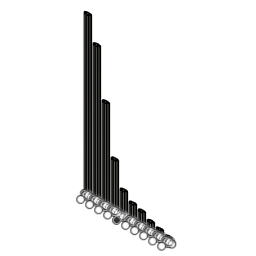
TT Clips 2020 v5 (Autodesk Fusion 360 design; units mm, degrees)
Autodesk Fusion 360 part; units mm, degrees
other "Mesh1"
sketch "Sketch1" plane through (0, 0, 0) normal (0, 0, 1) x (1, 0, 0)
  line L0 (-7.5, -1.2) -> (-7.5, 0)
  arc A0 (3.2, 0) -> (2, -1.2) centre (3.2, -1.2) ccw
  line L1 (3.2, -1.2) -> (7.5, -1.2)
  arc A1 (-6.7104, 1.1276) -> (-7.5, 0) centre (-6.3, 0) ccw
  line L2 (-2, -1.2) -> (-2, -4.3798)
  line L3 (2, -1.2) -> (2, -4.3798)
  arc A2 (-3.2, -3.4) -> (-2, -4.3798) centre (-3, -4.3798) ccw
  line L4 (-3.2, -3.4) -> (-3.2, -1.2)
  arc A3 (7.5, 0) -> (6.7104, 1.1276) centre (6.3, 0) ccw
  arc A4 (2, -4.3798) -> (3.2, -3.4) centre (3, -4.3798) ccw
  line L5 (7.5, -1.2) -> (7.5, 0)
  line L6 (6.3, 0) -> (3.2, 0)
  arc A5 (-2, -1.2) -> (-3.2, 0) centre (-3.2, -1.2) ccw
  line L7 (0, -6.5) -> (0, 3.9) construction
  line L8 (-3.2, -1.2) -> (-7.5, -1.2)
  line L9 (3.2, -3.4) -> (3.2, -1.2)
  line L10 (-6.3, 0) -> (-3.2, 0)
  arc A6 (6.7104, 1.1276) -> (-6.7104, 1.1276) centre (0, -17.3091) ccw
  arc A7 (6.3, 0) -> (-6.3, 0) centre (0, -16.1091) ccw
  line L11 (-80, -6.5) -> (-80, 3.9) construction
  arc A8 (-76.8, 0) -> (-78, -1.2) centre (-76.8, -1.2) ccw
  line L12 (-83.2, -3.4) -> (-83.2, -1.2)
  line L13 (-72.5, -1.2) -> (-72.5, 0)
  line L14 (-76.8, -3.4) -> (-76.8, -1.2)
  line L15 (-87.5, -1.2) -> (-87.5, 0)
  arc A9 (-78, -4.3798) -> (-76.8, -3.4) centre (-77, -4.3798) ccw
  line L16 (-82, -1.2) -> (-82, -4.3798)
  arc A10 (-86.7104, 1.1276) -> (-87.5, 0) centre (-86.3, 0) ccw
  line L17 (-86.3, 0) -> (-83.2, 0)
  line L18 (-78, -1.2) -> (-78, -4.3798)
  arc A11 (-82, -1.2) -> (-83.2, 0) centre (-83.2, -1.2) ccw
  arc A12 (-83.2, -3.4) -> (-82, -4.3798) centre (-83, -4.3798) ccw
  line L19 (-83.2, -1.2) -> (-87.5, -1.2)
  line L20 (-73.7, 0) -> (-76.8, 0)
  arc A13 (-73.2896, 1.1276) -> (-86.7104, 1.1276) centre (-80, -17.3091) ccw
  arc A14 (-73.7, 0) -> (-86.3, 0) centre (-80, -16.1091) ccw
  line L21 (-76.8, -1.2) -> (-72.5, -1.2)
  arc A15 (-72.5, 0) -> (-73.2896, 1.1276) centre (-73.7, 0) ccw
  line L22 (-60, -6.5) -> (-60, 3.9) construction
  arc A16 (-56.8, 0) -> (-58, -1.2) centre (-56.8, -1.2) ccw
  line L23 (-63.2, -3.4) -> (-63.2, -1.2)
  line L24 (-52.5, -1.2) -> (-52.5, 0)
  line L25 (-56.8, -3.4) -> (-56.8, -1.2)
  line L26 (-67.5, -1.2) -> (-67.5, 0)
  arc A17 (-58, -4.3798) -> (-56.8, -3.4) centre (-57, -4.3798) ccw
  line L27 (-62, -1.2) -> (-62, -4.3798)
  arc A18 (-66.7104, 1.1276) -> (-67.5, 0) centre (-66.3, 0) ccw
  line L28 (-66.3, 0) -> (-63.2, 0)
  line L29 (-58, -1.2) -> (-58, -4.3798)
  arc A19 (-62, -1.2) -> (-63.2, 0) centre (-63.2, -1.2) ccw
  arc A20 (-63.2, -3.4) -> (-62, -4.3798) centre (-63, -4.3798) ccw
  line L30 (-63.2, -1.2) -> (-67.5, -1.2)
  line L31 (-53.7, 0) -> (-56.8, 0)
  arc A21 (-53.2896, 1.1276) -> (-66.7104, 1.1276) centre (-60, -17.3091) ccw
  arc A22 (-53.7, 0) -> (-66.3, 0) centre (-60, -16.1091) ccw
  line L32 (-56.8, -1.2) -> (-52.5, -1.2)
  arc A23 (-52.5, 0) -> (-53.2896, 1.1276) centre (-53.7, 0) ccw
  line L33 (-40, -6.5) -> (-40, 3.9) construction
  arc A24 (-36.8, 0) -> (-38, -1.2) centre (-36.8, -1.2) ccw
  line L34 (-43.2, -3.4) -> (-43.2, -1.2)
  line L35 (-32.5, -1.2) -> (-32.5, 0)
  line L36 (-36.8, -3.4) -> (-36.8, -1.2)
  line L37 (-47.5, -1.2) -> (-47.5, 0)
  arc A25 (-38, -4.3798) -> (-36.8, -3.4) centre (-37, -4.3798) ccw
  line L38 (-42, -1.2) -> (-42, -4.3798)
  arc A26 (-46.7104, 1.1276) -> (-47.5, 0) centre (-46.3, 0) ccw
  line L39 (-46.3, 0) -> (-43.2, 0)
  line L40 (-38, -1.2) -> (-38, -4.3798)
  arc A27 (-42, -1.2) -> (-43.2, 0) centre (-43.2, -1.2) ccw
  arc A28 (-43.2, -3.4) -> (-42, -4.3798) centre (-43, -4.3798) ccw
  line L41 (-43.2, -1.2) -> (-47.5, -1.2)
  line L42 (-33.7, 0) -> (-36.8, 0)
  arc A29 (-33.2896, 1.1276) -> (-46.7104, 1.1276) centre (-40, -17.3091) ccw
  arc A30 (-33.7, 0) -> (-46.3, 0) centre (-40, -16.1091) ccw
  line L43 (-36.8, -1.2) -> (-32.5, -1.2)
  arc A31 (-32.5, 0) -> (-33.2896, 1.1276) centre (-33.7, 0) ccw
  line L44 (-20, -6.5) -> (-20, 3.9) construction
  arc A32 (-16.8, 0) -> (-18, -1.2) centre (-16.8, -1.2) ccw
  line L45 (-23.2, -3.4) -> (-23.2, -1.2)
  line L46 (-12.5, -1.2) -> (-12.5, 0)
  line L47 (-16.8, -3.4) -> (-16.8, -1.2)
  line L48 (-27.5, -1.2) -> (-27.5, 0)
  arc A33 (-18, -4.3798) -> (-16.8, -3.4) centre (-17, -4.3798) ccw
  line L49 (-22, -1.2) -> (-22, -4.3798)
  arc A34 (-26.7104, 1.1276) -> (-27.5, 0) centre (-26.3, 0) ccw
  line L50 (-26.3, 0) -> (-23.2, 0)
  line L51 (-18, -1.2) -> (-18, -4.3798)
  arc A35 (-22, -1.2) -> (-23.2, 0) centre (-23.2, -1.2) ccw
  arc A36 (-23.2, -3.4) -> (-22, -4.3798) centre (-23, -4.3798) ccw
  line L52 (-23.2, -1.2) -> (-27.5, -1.2)
  line L53 (-13.7, 0) -> (-16.8, 0)
  arc A37 (-13.2896, 1.1276) -> (-26.7104, 1.1276) centre (-20, -17.3091) ccw
  arc A38 (-13.7, 0) -> (-26.3, 0) centre (-20, -16.1091) ccw
  line L54 (-16.8, -1.2) -> (-12.5, -1.2)
  arc A39 (-12.5, 0) -> (-13.2896, 1.1276) centre (-13.7, 0) ccw
  line L55 (20, -6.5) -> (20, 3.9) construction
  arc A40 (23.2, 0) -> (22, -1.2) centre (23.2, -1.2) ccw
  line L56 (16.8, -3.4) -> (16.8, -1.2)
  line L57 (27.5, -1.2) -> (27.5, 0)
  line L58 (23.2, -3.4) -> (23.2, -1.2)
  line L59 (12.5, -1.2) -> (12.5, 0)
  arc A41 (22, -4.3798) -> (23.2, -3.4) centre (23, -4.3798) ccw
  line L60 (18, -1.2) -> (18, -4.3798)
  arc A42 (13.2896, 1.1276) -> (12.5, 0) centre (13.7, 0) ccw
  line L61 (13.7, 0) -> (16.8, 0)
  line L62 (22, -1.2) -> (22, -4.3798)
  arc A43 (18, -1.2) -> (16.8, 0) centre (16.8, -1.2) ccw
  arc A44 (16.8, -3.4) -> (18, -4.3798) centre (17, -4.3798) ccw
  line L63 (16.8, -1.2) -> (12.5, -1.2)
  line L64 (26.3, 0) -> (23.2, 0)
  arc A45 (26.7104, 1.1276) -> (13.2896, 1.1276) centre (20, -17.3091) ccw
  arc A46 (26.3, 0) -> (13.7, 0) centre (20, -16.1091) ccw
  line L65 (23.2, -1.2) -> (27.5, -1.2)
  arc A47 (27.5, 0) -> (26.7104, 1.1276) centre (26.3, 0) ccw
  line L66 (40, -6.5) -> (40, 3.9) construction
  arc A48 (43.2, 0) -> (42, -1.2) centre (43.2, -1.2) ccw
  line L67 (36.8, -3.4) -> (36.8, -1.2)
  line L68 (47.5, -1.2) -> (47.5, 0)
  line L69 (43.2, -3.4) -> (43.2, -1.2)
  line L70 (32.5, -1.2) -> (32.5, 0)
  arc A49 (42, -4.3798) -> (43.2, -3.4) centre (43, -4.3798) ccw
  line L71 (38, -1.2) -> (38, -4.3798)
  arc A50 (33.2896, 1.1276) -> (32.5, 0) centre (33.7, 0) ccw
  line L72 (33.7, 0) -> (36.8, 0)
  line L73 (42, -1.2) -> (42, -4.3798)
  arc A51 (38, -1.2) -> (36.8, 0) centre (36.8, -1.2) ccw
  arc A52 (36.8, -3.4) -> (38, -4.3798) centre (37, -4.3798) ccw
  line L74 (36.8, -1.2) -> (32.5, -1.2)
  line L75 (46.3, 0) -> (43.2, 0)
  arc A53 (46.7104, 1.1276) -> (33.2896, 1.1276) centre (40, -17.3091) ccw
  arc A54 (46.3, 0) -> (33.7, 0) centre (40, -16.1091) ccw
  line L76 (43.2, -1.2) -> (47.5, -1.2)
  arc A55 (47.5, 0) -> (46.7104, 1.1276) centre (46.3, 0) ccw
  line L77 (60, -6.5) -> (60, 3.9) construction
  arc A56 (63.2, 0) -> (62, -1.2) centre (63.2, -1.2) ccw
  line L78 (56.8, -3.4) -> (56.8, -1.2)
  line L79 (67.5, -1.2) -> (67.5, 0)
  line L80 (63.2, -3.4) -> (63.2, -1.2)
  line L81 (52.5, -1.2) -> (52.5, 0)
  arc A57 (62, -4.3798) -> (63.2, -3.4) centre (63, -4.3798) ccw
  line L82 (58, -1.2) -> (58, -4.3798)
  arc A58 (53.2896, 1.1276) -> (52.5, 0) centre (53.7, 0) ccw
  line L83 (53.7, 0) -> (56.8, 0)
  line L84 (62, -1.2) -> (62, -4.3798)
  arc A59 (58, -1.2) -> (56.8, 0) centre (56.8, -1.2) ccw
  arc A60 (56.8, -3.4) -> (58, -4.3798) centre (57, -4.3798) ccw
  line L85 (56.8, -1.2) -> (52.5, -1.2)
  line L86 (66.3, 0) -> (63.2, 0)
  arc A61 (66.7104, 1.1276) -> (53.2896, 1.1276) centre (60, -17.3091) ccw
  arc A62 (66.3, 0) -> (53.7, 0) centre (60, -16.1091) ccw
  line L87 (63.2, -1.2) -> (67.5, -1.2)
  arc A63 (67.5, 0) -> (66.7104, 1.1276) centre (66.3, 0) ccw
  line L88 (80, -6.5) -> (80, 3.9) construction
  arc A64 (83.2, 0) -> (82, -1.2) centre (83.2, -1.2) ccw
  line L89 (76.8, -3.4) -> (76.8, -1.2)
  line L90 (87.5, -1.2) -> (87.5, 0)
  line L91 (83.2, -3.4) -> (83.2, -1.2)
  line L92 (72.5, -1.2) -> (72.5, 0)
  arc A65 (82, -4.3798) -> (83.2, -3.4) centre (83, -4.3798) ccw
  line L93 (78, -1.2) -> (78, -4.3798)
  arc A66 (73.2896, 1.1276) -> (72.5, 0) centre (73.7, 0) ccw
  line L94 (73.7, 0) -> (76.8, 0)
  line L95 (82, -1.2) -> (82, -4.3798)
  arc A67 (78, -1.2) -> (76.8, 0) centre (76.8, -1.2) ccw
  arc A68 (76.8, -3.4) -> (78, -4.3798) centre (77, -4.3798) ccw
  line L96 (76.8, -1.2) -> (72.5, -1.2)
  line L97 (86.3, 0) -> (83.2, 0)
  arc A69 (86.7104, 1.1276) -> (73.2896, 1.1276) centre (80, -17.3091) ccw
  arc A70 (86.3, 0) -> (73.7, 0) centre (80, -16.1091) ccw
  line L98 (83.2, -1.2) -> (87.5, -1.2)
  arc A71 (87.5, 0) -> (86.7104, 1.1276) centre (86.3, 0) ccw
  line L99 (100, -6.5) -> (100, 3.9) construction
  arc A72 (103.2, 0) -> (102, -1.2) centre (103.2, -1.2) ccw
  line L100 (96.8, -3.4) -> (96.8, -1.2)
  line L101 (107.5, -1.2) -> (107.5, 0)
  line L102 (103.2, -3.4) -> (103.2, -1.2)
  line L103 (92.5, -1.2) -> (92.5, 0)
  arc A73 (102, -4.3798) -> (103.2, -3.4) centre (103, -4.3798) ccw
  line L104 (98, -1.2) -> (98, -4.3798)
  arc A74 (93.2896, 1.1276) -> (92.5, 0) centre (93.7, 0) ccw
  line L105 (93.7, 0) -> (96.8, 0)
  line L106 (102, -1.2) -> (102, -4.3798)
  arc A75 (98, -1.2) -> (96.8, 0) centre (96.8, -1.2) ccw
  arc A76 (96.8, -3.4) -> (98, -4.3798) centre (97, -4.3798) ccw
  line L107 (96.8, -1.2) -> (92.5, -1.2)
  line L108 (106.3, 0) -> (103.2, 0)
  arc A77 (106.7104, 1.1276) -> (93.2896, 1.1276) centre (100, -17.3091) ccw
  arc A78 (106.3, 0) -> (93.7, 0) centre (100, -16.1091) ccw
  line L109 (103.2, -1.2) -> (107.5, -1.2)
  arc A79 (107.5, 0) -> (106.7104, 1.1276) centre (106.3, 0) ccw
  point P0 (0, -16.1091)
  point P1 (-80, 0)
  point P2 (-80, 0)
  point P3 (-80, 0)
  point P4 (-60, 0)
  point P5 (-60, 0)
  point P6 (-60, 0)
  point P7 (-40, 0)
  point P8 (-40, 0)
  point P9 (-40, 0)
  point P10 (-20, 0)
  point P11 (-20, 0)
  point P12 (-20, 0)
  point P13 (20, 0)
  point P14 (20, 0)
  point P15 (20, 0)
  point P16 (40, 0)
  point P17 (40, 0)
  point P18 (40, 0)
  point P19 (60, 0)
  point P20 (60, 0)
  point P21 (60, 0)
  point P22 (80, 0)
  point P23 (80, 0)
  point P24 (80, 0)
  point P25 (100, 0)
  point P26 (100, 0)
  point P27 (100, 0)
  dimension "d3" = 1.2
  dimension "d8" = 20
  dimension "d9" = 0
  constraint vertical L7
  constraint symmetric A2.start A4.end L7
  constraint symmetric L2.end L3.end L7
  constraint symmetric A2 A4 L7
  constraint tangent A1 A6
  constraint coincident P0 A7.centre
  measures "d3" distance of A6.centre P0
extrude "Extrude2" add sketch "Sketch1" along normal blind 50 contours L0 A0 L1 A1 L2 L3 A2 L4 A3 A4 L5 L6 A5 L8 L9 L10 A6 A7 makes body 1
extrude "Extrude3" add sketch "Sketch1" along normal blind 10 separate body contours A72 L100 L101 L102 L103 A73 L104 A74 L105 L106 A75 A76 L107 L108 A77 A78 L109 A79 makes body 2
extrude "Extrude4" add sketch "Sketch1" along normal blind 15 separate body contours A64 L89 L90 L91 L92 A65 L93 A66 L94 L95 A67 A68 L96 L97 A69 A70 L98 A71 makes body 3
extrude "Extrude5" add sketch "Sketch1" along normal blind 20 separate body contours A56 L78 L79 L80 L81 A57 L82 A58 L83 L84 A59 A60 L85 L86 A61 A62 L87 A63 makes body 4
extrude "Extrude6" add sketch "Sketch1" along normal blind 30 separate body contours A48 L67 L68 L69 L70 A49 L71 A50 L72 L73 A51 A52 L74 L75 A53 A54 L76 A55 makes body 5
extrude "Extrude7" add sketch "Sketch1" along normal blind 35 separate body contours A40 L56 L57 L58 L59 A41 L60 A42 L61 L62 A43 A44 L63 L64 A45 A46 L65 A47 makes body 6
extrude "Extrude8" add sketch "Sketch1" along normal blind 100 separate body contours A32 L45 L46 L47 L48 A33 L49 A34 L50 L51 A35 A36 L52 L53 A37 A38 L54 A39 makes body 7
extrude "Extrude9" add sketch "Sketch1" along normal blind 200 separate body contours A24 L34 L35 L36 L37 A25 L38 A26 L39 L40 A27 A28 L41 L42 A29 A30 L43 A31 makes body 8
extrude "Extrude10" add sketch "Sketch1" along normal blind 300 separate body contours A16 L23 L24 L25 L26 A17 L27 A18 L28 L29 A19 A20 L30 L31 A21 A22 L32 A23 makes body 9
extrude "Extrude11" add sketch "Sketch1" along normal blind 350 separate body contours A8 L12 L13 L14 L15 A9 L16 A10 L17 L18 A11 A12 L19 L20 A13 A14 L21 A15 makes body 10
named bodies: "50", "10", "15", "20", "30", "35", "100", "200", "300", "350"
